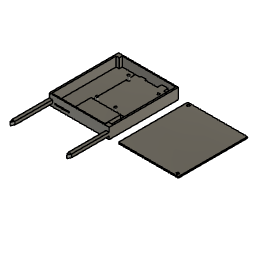
soilcase v2 (Autodesk Fusion 360 design; units mm, degrees)
Autodesk Fusion 360 part; units mm, degrees
note: some values were not read from the file. Chosen so that the rebuilt part matches the saved one: which bodies a step acts on; which face or edge a step refers to.
sketch "Sketch1" plane through (0, 0, 0) normal (0, 0, 1) x (1, 0, 0)
  line L0 (0, 70) -> (95, 70)
  line L1 (95, 70) -> (95, -40)
  line L2 (95, -40) -> (0, -40)
  line L3 (0, -40) -> (0, 70)
  dimension "d1" = 95
  dimension "d2" = 110
  constraint horizontal L0
  constraint vertical L1
  constraint horizontal L2
  constraint vertical L3
  measures "d1" distance of L0.start L0.end
  measures "d2" distance of L0.start L2.end
extrude "Extrude1" add sketch "Sketch1" along normal blind 17 makes body 1
sketch "Sketch2" plane through (0, 0, 17) normal (0, 0, 1) x (-1, 0, 0)
  line L0 (0, 40) -> (-95, 40)
  line L1 (-95, 40) -> (-95, -70)
  line L2 (-95, -70) -> (0, -70)
  line L3 (0, -70) -> (0, 40)
  line L4 (-2.4577, -68.4846) -> (-92.4577, -68.4846)
  line L5 (-92.4577, -68.4846) -> (-92.4577, 38.5154)
  line L6 (-92.4577, 38.5154) -> (-2.4577, 38.5154)
  line L7 (-2.4577, 38.5154) -> (-2.4577, -68.4846)
  dimension "d5" = 90
  dimension "d6" = 107
  constraint horizontal L4
  constraint vertical L5
  constraint horizontal L6
  constraint vertical L7
  measures "d5" distance of L4.start L4.end
  measures "d6" distance of L4.start L6.end
extrude "Extrude2" cut sketch "Sketch2" against normal blind 1.5 contours L4 L5 L6 L7 bodies 1
box "BoxPrimitive1" add length 77 width 55 height 10 placed x (0, -1, 0) y (1, 0, 0) z (0, 0, 1) at (150, 60, 0) separate body makes body 2
sketch "Sketch4" plane through (0, 0, 10) normal (0, 0, 1) x (-1, 0, 0)
  line L0 (-150, 17) -> (-205, 17)
  line L1 (-205, 17) -> (-205, -60)
  line L2 (-205, -60) -> (-150, -60)
  line L3 (-150, -60) -> (-150, 17)
  line L4 (-150, 14.0052) -> (-152, 14.0052)
  line L5 (-152, 14.0052) -> (-154.9948, 17)
  line L6 (-154.9948, 17) -> (-187.9948, 17)
  line L7 (-187.9948, 17) -> (-189.9555, 13.9808)
  line L8 (-187.9948, 17) -> (-184.3948, 17) construction
  line L9 (-189.9555, 13.9808) -> (-205, 13.9808)
  dimension "d14" = 135
  dimension "d15" = 33
  dimension "d16" = 123
  dimension "d17" = 3.6
  constraint coincident L3 L4.start
  constraint perpendicular L3 L4
  constraint coincident L0 L5.end
  constraint parallel L0 L6
  constraint horizontal L8
  constraint coincident L1 L9.end
  constraint perpendicular L1 L9
  measures "d14" angle of L4 L5
  measures "d15" distance of L5.end L6.end
  measures "d16" angle of L7 L8
  measures "d17" distance of L6.end L7.end
extrude "Extrude3" cut sketch "Sketch4" against normal blind 10 contours L0 L3 L4 L5 | L0 L1 L7 L9 bodies 2
sketch "Sketch5" plane through (0, 0, 10) normal (0, 0, 1) x (-1, 0, 0)
  line L0 (-187.9948, 17) -> (-189.9555, 13.9808)
  line L1 (-189.9555, 13.9808) -> (-205, 13.9808)
  line L2 (-205, 13.9808) -> (-205, -60)
  line L3 (-205, -60) -> (-150, -60)
  line L4 (-150, -60) -> (-150, 14.0052)
  line L5 (-150, 14.0052) -> (-152, 14.0052)
  line L6 (-152, 14.0052) -> (-154.9948, 17)
  line L7 (-154.9948, 17) -> (-187.9948, 17)
  line L8 (-205, -52.9686) -> (-195, -52.9686)
  line L9 (-195, -52.9686) -> (-195, -60)
  line L10 (-195, -60) -> (-185, -60)
  line L11 (-185, -60) -> (-185, -52.9686)
  line L12 (-185, -52.9686) -> (-165, -52.9686)
  line L13 (-165, -52.9686) -> (-165, -55)
  line L14 (-165, -55) -> (-157, -55)
  line L15 (-157, -55) -> (-157, -52.9686)
  line L16 (-157, -52.9686) -> (-150, -52.9686)
  dimension "d20" = 20
  constraint coincident L2 L8.start
  constraint perpendicular L2 L8
  constraint coincident L3 L9.end
  constraint perpendicular L3 L9
  constraint coincident L3 L10.end
  constraint perpendicular L9 L10
  constraint perpendicular L10 L11
  constraint perpendicular L4 L12
  constraint perpendicular L12 L13
  constraint perpendicular L13 L14
  constraint perpendicular L14 L15
  constraint coincident L4 L16.end
  constraint perpendicular L4 L16
  measures "d20" distance of L11.end L12.end
extrude "Extrude4" cut sketch "Sketch5" against normal blind 10 contours L2 L3 L8 L9 | L3 L4 L11 L12 L13 L14 L15 L16 bodies 2
copy_body "Body->Comp1" bodies 1 removing the originals makes body 3 in component "Case"
copy_body "Body->Comp2" bodies 2 removing the originals makes body 4 in component "UNO"
extrude "Extrude1'" cut 1 faces at (32.4577, 32.8179, 15.5) along direction (0, 0, -1) blind 13.5 on bodies 3 bodies 3 in component "Case"
hole "Hole1" at (201.9832, 37.725, 10) direction (0, 0, -1) diameter 4 depth 14 tip angle 118 bodies 4 in component "UNO"
hole "Hole2" at (152.3342, 39.8592, 10) direction (0, 0, -1) diameter 4 depth 14 tip angle 118 bodies 4 in component "UNO"
hole "Hole3" at (156.3427, -14.6411, 10) direction (0, 0, -1) diameter 4 depth 14 tip angle 118 bodies 4 in component "UNO"
hole "Hole4" at (185.8605, -14.7534, 10) direction (0, 0, -1) diameter 4 depth 14 tip angle 118 bodies 4 in component "UNO"
box "BoxPrimitive2" add length 25 width 47 height 1.6 placed x (0, -1, 0) y (1, 0, 0) z (0, 0, 1) at (98, 50, 0) separate body makes body 5
extrude "Extrude5" add 1 faces at (129.3333, 41.6667, 1.6) along direction (0, 0, 1) blind 14.4 on bodies 5 bodies 5
move_body "Move1" bodies 5 to x (1, 0, 0) y (0, 1, 0) z (0, 0, 1) at (-52.9645, -63.0783, -6)
move_body "Move1'" bodies 4 to x (1, 0, 0) y (0, 1, 0) z (0, 0, 1) at (-113.6474, 5.8554, 0) in component "UNO"
move_body "Move2" bodies 4 to x (1, 0, 0) y (0, 1, 0) z (0, 0, 1) at (0.5323, 0, 0) in component "UNO"
move_body "Move2'" bodies 5 to x (1, 0, 0) y (0, 1, 0) z (0, 0, 1) at (0, 0, 6)
move_body "Move3" bodies 5 to x (1, 0, 0) y (0, 1, 0) z (0, 0, 1) at (-0.2649, 0.5329, 0.0058)
move_body "Move3'" bodies 4 to x (1, 0, 0) y (0, 1, 0) z (0, 0, 1) at (-0.5286, 1.5981, 0.0116) in component "UNO"
copy_body "Body->Comp3" bodies 5 removing the originals makes body 6 in component "Battery"
sketch "Sketch7" plane through (0, -40, 0) normal (0, -1, 0) x (1, 0, 0)
  line L0 (0, 0) -> (95, 0)
  line L1 (95, 0) -> (95, 17)
  line L2 (95, 17) -> (0, 17)
  line L3 (0, 17) -> (0, 0)
  line L4 (8.4897, 5) -> (31.4897, 5)
  line L5 (31.4897, 5) -> (31.4897, 6.5)
  line L6 (31.4897, 6.5) -> (8.4897, 6.5)
  line L7 (8.4897, 6.5) -> (8.4897, 5)
  dimension "d44" = 23
  dimension "d45" = 1.5
  constraint horizontal L4
  constraint vertical L5
  constraint horizontal L6
  constraint vertical L7
  measures "d44" distance of L4.start L4.end
  measures "d45" distance of L4.start L6.end
extrude "Extrude2'" cut sketch "Sketch7" against normal blind 10 contours L4 L5 L6 L7 bodies 3 in component "Case"
sketch "Sketch8" plane through (0, -40, 0) normal (0, -1, 0) x (1, 0, 0)
  line L0 (31.4897, 5) -> (8.4897, 5)
  line L1 (8.4897, 5) -> (8.4897, 6.5)
  line L2 (8.4897, 6.5) -> (31.4897, 6.5)
  line L3 (31.4897, 6.5) -> (31.4897, 5)
  line L4 (0, 0) -> (95, 0)
  line L5 (95, 0) -> (95, 17)
  line L6 (95, 17) -> (0, 17)
  line L7 (0, 17) -> (0, 0)
  line L8 (0, 10) -> (5, 10)
  line L9 (5, 10) -> (5, 5)
  line L10 (5, 5) -> (0, 5)
  line L11 (0, 5) -> (0, 10)
  constraint horizontal L8
  constraint vertical L9
  constraint horizontal L10
  constraint vertical L11
  constraint coincident L7 L8.start
extrude "Extrude3'" add sketch "Sketch8" along normal blind 60 contours L7 L8 L9 L10 L11 bodies 3 in component "Case"
sketch "Sketch9" plane through (0, -40, 0) normal (0, -1, 0) x (1, 0, 0)
  line L0 (0, 10) -> (5, 10)
  line L1 (5, 10) -> (5, 5)
  line L2 (5, 5) -> (0, 5)
  line L3 (0, 5) -> (0, 0)
  line L4 (0, 0) -> (95, 0)
  line L5 (95, 0) -> (95, 17)
  line L6 (95, 17) -> (0, 17)
  line L7 (0, 17) -> (0, 10)
  line L8 (31.4897, 5) -> (8.4897, 5)
  line L9 (8.4897, 5) -> (8.4897, 6.5)
  line L10 (8.4897, 6.5) -> (31.4897, 6.5)
  line L11 (31.4897, 6.5) -> (31.4897, 5)
  line L12 (95, 10.0559) -> (90, 10.0559)
  line L13 (90, 10.0559) -> (90, 5)
  line L14 (90, 5) -> (95, 5)
  line L15 (95, 5) -> (95, 10.0559)
  constraint horizontal L12
  constraint vertical L13
  constraint horizontal L14
  constraint vertical L15
  constraint coincident L5 L12.start
extrude "Extrude4'" add sketch "Sketch9" along normal blind 60 contours L5 L12 L13 L14 L15 bodies 3 in component "Case"
sketch "Sketch10" plane through (0, 0, 0) normal (0, 0, 1) x (1, 0, 0)
sketch "Sketch11" plane through (0, 0, 0) normal (0, 0, 1) x (1, 0, 0)
  line L0 (35, -65) -> (40, -65)
  line L1 (40, -65) -> (37.5, -70.0077)
  line L2 (37.5, -70.0077) -> (35, -65)
  constraint horizontal L0
extrude "Extrude6" add sketch "Sketch11" along normal blind 5 separate body makes body 7
copy_body "CopyPasteBodies1" bodies 7 makes body 8
move_body "Move4" bodies 8 to x (1, 0, 0) y (0, 1, 0) z (0, 0, 1) at (10.0748, -0.1782, -0.1413)
move_body "Move5" bodies 7 to x (1, 0, 0) y (0, 1, 0) z (0, 0, 1) at (-33.4305, -17.0553, -10.3398)
move_body "Move6" bodies 7 to x (1, 0, 0) y (0, 1, 0) z (0, 0, 1) at (-1.6067, -18.5396, 15.585)
move_body "Move7" bodies 7 to x (1, 0, 0) y (0, 1, 0) z (0, 0, 1) at (0, 0.5925, 0)
combine "Combine1" operation add target body 3 tool bodies 7 makes body 9 at (4.1294, -101.6717, 8.5785) in component "Case"
move_body "Move8" bodies 8 to x (1, 0, 0) y (0, 1, 0) z (0, 0, 1) at (44.9335, -34.8605, 5.2)
combine "Combine2" operation add target body 3 tool bodies 8 makes body 10 at (94.1749, -101.7079, 6.7254) in component "Case"
move_body "Move1''" bodies 6 to x (1, 0, 0) y (0, 1, 0) z (0, 0, 1) at (-6.0243, 0, 0) in component "Battery"
sketch "Sketch12" plane through (0, 0, 2) normal (0, 0, 1) x (-1, 0, 0)
  line L0 (-2.4577, 38.5154) -> (-92.4577, 38.5154)
  line L1 (-92.4577, 38.5154) -> (-92.4577, -68.4846)
  line L2 (-92.4577, -68.4846) -> (-2.4577, -68.4846)
  line L3 (-2.4577, -68.4846) -> (-2.4577, 38.5154)
  line L4 (-2.4577, -68.4846) -> (-7.4577, -68.4846)
  line L5 (-7.4577, -68.4846) -> (-7.4577, -63.4846)
  line L6 (-7.4577, -63.4846) -> (-2.4577, -63.4846)
  line L7 (-2.4577, -63.4846) -> (-2.4577, -68.4846)
  dimension "d54" = 5
  dimension "d55" = 5
  constraint horizontal L4
  constraint vertical L5
  constraint horizontal L6
  constraint vertical L7
  constraint coincident L2.end L3.start
  measures "d54" distance of L2.end L4.end
  measures "d55" distance of L2.end L6.end
extrude "Extrude5'" add sketch "Sketch12" along normal blind 15 contours L2 L3 L4 L5 L6 L7 bodies 3 in component "Case"
sketch "Sketch13" plane through (0, 0, 2) normal (0, 0, 1) x (-1, 0, 0)
  line L0 (-7.4577, -68.4846) -> (-7.4577, -63.4846)
  line L1 (-7.4577, -63.4846) -> (-2.4577, -63.4846)
  line L2 (-2.4577, -63.4846) -> (-2.4577, 38.5154)
  line L3 (-2.4577, 38.5154) -> (-92.4577, 38.5154)
  line L4 (-92.4577, 38.5154) -> (-92.4577, -68.4846)
  line L5 (-92.4577, -68.4846) -> (-7.4577, -68.4846)
  line L6 (-92.4577, 38.5154) -> (-87.4577, 38.5154)
  line L7 (-87.4577, 38.5154) -> (-87.4577, 33.5154)
  line L8 (-87.4577, 33.5154) -> (-92.4577, 33.5154)
  line L9 (-92.4577, 33.5154) -> (-92.4577, 38.5154)
  dimension "d58" = 5
  dimension "d59" = 5
  constraint horizontal L6
  constraint vertical L7
  constraint horizontal L8
  constraint vertical L9
  constraint coincident L3.end L4.start
  measures "d58" distance of L3.end L6.end
  measures "d59" distance of L3.end L8.end
extrude "Extrude6'" add sketch "Sketch13" along normal blind 15 contours L3 L4 L6 L7 L8 L9 bodies 3 in component "Case"
sketch "Sketch14" plane through (0, 0, 2) normal (0, 0, 1) x (-1, 0, 0)
  line L0 (-87.4577, 38.5154) -> (-87.4577, 33.5154)
  line L1 (-87.4577, 33.5154) -> (-92.4577, 33.5154)
  line L2 (-92.4577, 33.5154) -> (-92.4577, -68.4846)
  line L3 (-92.4577, -68.4846) -> (-7.4577, -68.4846)
  line L4 (-7.4577, -68.4846) -> (-7.4577, -63.4846)
  line L5 (-7.4577, -63.4846) -> (-2.4577, -63.4846)
  line L6 (-2.4577, -63.4846) -> (-2.4577, 38.5154)
  line L7 (-2.4577, 38.5154) -> (-87.4577, 38.5154)
  circle A0 centre (-72.2, 7.3) radius 1.9007
extrude "Extrude7" add sketch "Sketch14" along normal blind 15 contours A0 bodies 3 in component "Case"
sketch "Sketch15" plane through (0, 0, 2) normal (0, 0, 1) x (-1, 0, 0)
  circle A0 centre (-72.2, 7.3) radius 1.9007
  line L0 (-87.4577, 38.5154) -> (-87.4577, 33.5154)
  line L1 (-87.4577, 33.5154) -> (-92.4577, 33.5154)
  line L2 (-92.4577, 33.5154) -> (-92.4577, -68.4846)
  line L3 (-92.4577, -68.4846) -> (-7.4577, -68.4846)
  line L4 (-7.4577, -68.4846) -> (-7.4577, -63.4846)
  line L5 (-7.4577, -63.4846) -> (-2.4577, -63.4846)
  line L6 (-2.4577, -63.4846) -> (-2.4577, 38.5154)
  line L7 (-2.4577, 38.5154) -> (-87.4577, 38.5154)
  circle A1 centre (-42.7, 7.2) radius 1.9007
extrude "Extrude8" add sketch "Sketch15" along normal blind 15 contours A1 bodies 3 in component "Case"
sketch "Sketch16" plane through (0, 0, 2) normal (0, 0, 1) x (-1, 0, 0)
  circle A0 centre (-42.7, 7.2) radius 1.9007
  circle A1 centre (-72.2, 7.3) radius 1.9007
  line L0 (-87.4577, 38.5154) -> (-87.4577, 33.5154)
  line L1 (-87.4577, 33.5154) -> (-92.4577, 33.5154)
  line L2 (-92.4577, 33.5154) -> (-92.4577, -68.4846)
  line L3 (-92.4577, -68.4846) -> (-7.4577, -68.4846)
  line L4 (-7.4577, -68.4846) -> (-7.4577, -63.4846)
  line L5 (-7.4577, -63.4846) -> (-2.4577, -63.4846)
  line L6 (-2.4577, -63.4846) -> (-2.4577, 38.5154)
  line L7 (-2.4577, 38.5154) -> (-87.4577, 38.5154)
  circle A2 centre (-38.7, -47.3) radius 1.9
extrude "Extrude9" add sketch "Sketch16" along normal blind 15 contours A2 bodies 3 in component "Case"
sketch "Sketch17" plane through (0, 0, 2) normal (0, 0, 1) x (-1, 0, 0)
  circle A0 centre (-38.7, -47.3) radius 1.9
  circle A1 centre (-42.7, 7.2) radius 1.9007
  circle A2 centre (-72.2, 7.3) radius 1.9007
  line L0 (-87.4577, 38.5154) -> (-87.4577, 33.5154)
  line L1 (-87.4577, 33.5154) -> (-92.4577, 33.5154)
  line L2 (-92.4577, 33.5154) -> (-92.4577, -68.4846)
  line L3 (-92.4577, -68.4846) -> (-7.4577, -68.4846)
  line L4 (-7.4577, -68.4846) -> (-7.4577, -63.4846)
  line L5 (-7.4577, -63.4846) -> (-2.4577, -63.4846)
  line L6 (-2.4577, -63.4846) -> (-2.4577, 38.5154)
  line L7 (-2.4577, 38.5154) -> (-87.4577, 38.5154)
  circle A3 centre (-88.35, -45.2) radius 1.9007
extrude "Extrude10" add sketch "Sketch17" along normal blind 15 contours A3 bodies 3 in component "Case"
box "BoxPrimitive3" add length 110 width 95 height 2 placed x (0, -1, 0) y (1, 0, 0) z (0, 0, 1) at (110, 70, 2) separate body makes body 11
hole "Hole1'" at (114.9345, 66.1742, 4) direction (0, 0, -1) diameter 4 depth 4 tip angle 180 bodies 11
hole "Hole2'" at (200.1174, -36.1123, 4) direction (0, 0, -1) diameter 4 depth 4 tip angle 180 bodies 11
copy_body "Body->Comp4" bodies 11 removing the originals makes body 12 in component "Component"
component "Case" placed x (1, 0, 0) y (0, 1, 0) z (0, 0, 1) at (0, 0, 0)
component "UNO" placed x (1, 0, 0) y (0, 1, 0) z (0, 0, 1) at (0, 0, 0)
component "Battery" placed x (1, 0, 0) y (0, 1, 0) z (0, 0, 1) at (0, 0, 0)
component "Component" placed x (1, 0, 0) y (0, 1, 0) z (0, 0, 1) at (0, 0, 0)
